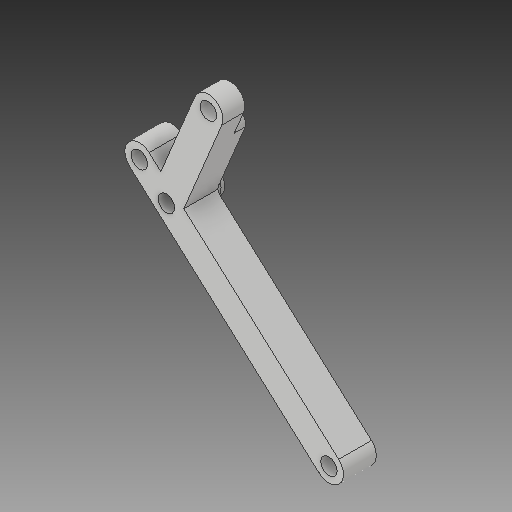
# Autodesk Inventor part: MasiveTriangle
Saved by Autodesk Inventor 2017 (Build 210142000, 142)
## iProperties
Created: 2020-09-06
Part Number: MasiveTriangle
Material: Generic
Document SubType Name: Modeling
Designer: agustin
Density: 1 g/cm^3
Appearance: Default
Author: agustin
Autodesk Inventor part; units mm, degrees
ref_plane "YZ Plane" through (0, 0, 0) normal (1, 0, 0) x (0, 1, 0)
ref_plane "XZ Plane" through (0, 0, 0) normal (0, 1, 0) x (-1, 0, 0)
ref_plane "XY Plane" through (0, 0, 0) normal (0, 0, 1) x (1, 0, 0)
sketch "Sketch1" plane through (0, 0, 0) normal (0, 0, 1) x (1, 0, 0)
  circle A0 centre (28.4266, -32.3962) radius 2.25 projected
  circle A1 centre (-23.5739, 14.4648) radius 2.25 projected
  circle A2 centre (-16.1457, 7.7699) radius 2.25 projected
  circle A3 centre (-4.6396, 35.4757) radius 2.25 projected
  line L0 (28.4266, -32.3962) -> (-23.5739, 14.4648) construction
  line L1 (-26.2516, 11.4934) -> (25.7488, -35.3676)
  arc A4 (25.7488, -35.3676) -> (31.1043, -29.4247) centre (28.4266, -32.3962) ccw
  arc A5 (-20.8961, 17.4363) -> (-26.2516, 11.4934) centre (-23.5739, 14.4648) ccw
  line L2 (-16.1457, 7.7699) -> (-4.6396, 35.4757) construction
  line L3 (-11.3665, 8.8485) -> (-0.9455, 33.9415)
  arc A6 (-18.877, 4.8476) -> (-18.769, 4.7503) centre (-16.1457, 7.7699) ccw
  arc A7 (-0.9455, 33.9415) -> (-8.3337, 37.0098) centre (-4.6396, 35.4757) ccw
  line L4 (-8.3337, 37.0098) -> (-17.6699, 14.529)
  line L5 (-19.2971, 10.6108) -> (-19.8398, 9.3041)
  line L6 (31.1043, -29.4247) -> (-11.3665, 8.8485)
  line L7 (-17.6699, 14.529) -> (-20.8961, 17.4363)
  point P0 (0, 0)
  point P1 (2.4263, -8.9657)
  point P2 (-10.3926, 21.6228)
  dimension "d0" = 8
  dimension "d1" = 8
  constraints: 20 end point, 12 tangent, 8 point on circle, 4 centre point, 4 parallel, 3 point on line, 2 midpoint
  measures "d0" diameter of A5
  measures "d1" diameter of A7
extrude "Extrusion1" add sketch "Sketch1" along normal blind 9
sketch "Sketch2" plane through (0, 0, 0) normal (0, 0, -1) x (-1, 0, 0)
  circle A0 centre (16.1457, 7.7699) radius 2.25 projected
  circle A1 centre (16.1457, 7.7699) radius 2.25
  circle A2 centre (16.1457, 7.7699) radius 4
  point P0 (0, 0)
  dimension "d4" = 8
  constraints: 2 centre point, 2 coincident
  measures "d4" diameter of A2
extrude "Extrusion2" add sketch "Sketch2" along normal blind 3
sketch "Sketch5" plane through (0, 0, 0) normal (0, 0, -1) x (-1, 0, 0)
  circle A0 centre (4.6396, 35.4757) radius 2.25 projected
  circle A1 centre (4.6396, 35.4757) radius 5
  point P0 (0, 0)
  dimension "d16" = 10
  constraints: 1 centre point, 1 coincident
  measures "d16" diameter of A1
extrude "Extrusion5" cut sketch "Sketch5" against normal blind 3
fillet "Fillet1" radius 2 4 edges at (-12.5061, 9.4292, 0) (-19.8148, 6.177, 0) (-2.0961, 31.171, 1.5) (-9.4843, 34.2393, 1.5)
scale "Scale1" factors (0.5, 0.5, 0.5) then translate (-0.1257, -5.9686, 4.5) bodies 1
body "Solid1"
